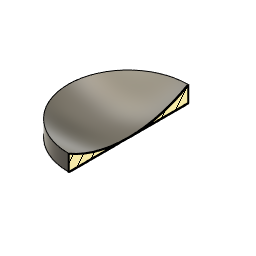
sphere_holder v8 (Autodesk Fusion 360 design; units mm, degrees)
Autodesk Fusion 360 part; units mm, degrees
sphere "SpherePrimitive1" add diameter 80 placed x (1, 0, 0) y (0, 0, -1) z (0, 1, 0) at (0, 0, 0) makes body 1 in component "sphere"
ref_plane "WorkPlane1" through (0, -40, 0) normal (0, 1, 0) x (0, 0, 1) in component "holder"
sketch "Sketch1" plane through (0, -40, 0) normal (0, 1, 0) x (1, 0, 0) in component "holder"
  circle A0 centre (0, 0) radius 20
  dimension "d3" = 40
  constraint coincident A0.centre origin
  measures "d3" diameter of A0
extrude "Extrude1" add sketch "Sketch1" along normal blind 10 separate body makes body 2 in component "holder"
combine "Combine1" operation cut target body 2 tool bodies 1 keep tools in component "holder"
ref_plane "WorkPlane1" through (0, -40, 0) normal (0, 1, 0) x (0, 0, 1) in component "holder (1)"
sketch "Sketch1 (2)" plane through (0, -40, 0) normal (0, 1, 0) x (1, 0, 0) in component "holder (1)"
  circle A0 centre (0, 0) radius 20
  dimension "d3_1" = 40
  constraint coincident A0.centre origin
  measures "d3_1" diameter of A0
extrude "Extrude1'" add sketch "Sketch1 (2)" along normal blind 10 separate body makes body 3 in component "holder (1)"
combine "Combine1'" operation cut target body 3 tool bodies 1 keep tools in component "holder (1)"
component "sphere" placed x (1, 0, 0) y (0, 1, 0) z (0, 0, 1) at (0, 0, 0)
component "holder" placed x (1, 0, 0) y (0, 1, 0) z (0, 0, 1) at (0, 0, 0)
component "holder (1)" placed x (1, 0, 0) y (0, 1, 0) z (0, 0, 1) at (0, 0, 0)
